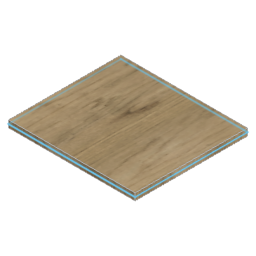
_Project Panel (Sliding Platform).133bd67c-09e4-451d-a58f-389c6de2ee63 (Autodesk Fusion 360 design; units mm, degrees)
Autodesk Fusion 360 part; units mm, degrees
sketch "sketch 295" plane through (0, 0, 37.546) normal (0, 0, 1) x (1, 0, 0)
  line L0 (308.6682, 292.5515) -> (648.5481, 292.5515)
  line L1 (308.6682, 292.5515) -> (648.5481, 292.5515)
  line L2 (308.6682, -9.1484) -> (308.6682, 292.5515)
  line L3 (648.5481, -9.1484) -> (308.6682, -9.1484)
  line L4 (648.5481, -9.1484) -> (308.6682, -9.1484)
  line L5 (648.5481, 292.5515) -> (648.5481, -9.1484)
extrude "Extrude1" add sketch "sketch 295" along normal mid plane 19.04
